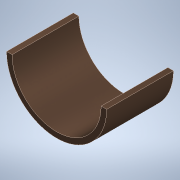
# Autodesk Inventor part: Верхняя часть коренного подшипника
Saved by Autodesk Inventor 2021 (Build 250183000, 183)
## iProperties
Created: 2020-12-05
Part Number: Верхняя часть коренного подшипника
Material: Бронза, литейная
Document SubType Name: Modeling
Designer: Тимоха
Mass: 2835.31 g
Surface Area: 719.857 cm^2
Volume: 319.652 cm^3
Density: 8.87 g/cm^3
Appearance: Бронза - сатинированная
Author: Тимоха
Autodesk Inventor part; units mm, degrees
ref_plane "YZ Plane" through (0, 0, 0) normal (1, 0, 0) x (0, 1, 0)
ref_plane "XZ Plane" through (0, 0, 0) normal (0, 1, 0) x (-1, 0, 0)
ref_plane "XY Plane" through (0, 0, 0) normal (0, 0, 1) x (1, 0, 0)
sketch "Эскиз1" plane through (0, 0, 0) normal (0, 0, 1) x (1, 0, 0)
  circle A0 centre (0, 0) radius 80
  circle A1 centre (0, 0) radius 90
  line L0 (-90, 0) -> (90, 0)
  point P0 (-80, 0)
  point P1 (80, 0)
  dimension "d0" = 160
  dimension "d1" = 180
  constraints: 2 centre point, 2 coincident, 2 end point, 2 point on circle, 1 horizontal
  measures "d0" diameter of A0
  measures "d1" diameter of A1
extrude "Выдавливание1" add sketch "Эскиз1" along normal blind 120 contours L0 A1 A0 picked at (54.1763, -63.1025)
